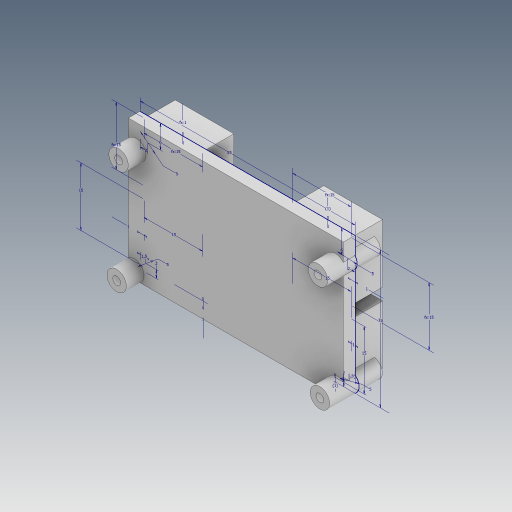
# Autodesk Inventor part: Attacco scheda 2
Saved by Autodesk Inventor 2023.2 (Build 272271000, 271)
## iProperties
Created: 2022-11-27
Part Number: Attacco scheda 2
Material: Generico
Document SubType Name: Modeling
Designer: daler
Density: 1 g/cm^3
Appearance: Default
Author: daler
Autodesk Inventor part; units mm, degrees
ref_plane "YZ Plane" through (0, 0, 0) normal (1, 0, 0) x (0, 1, 0)
ref_plane "XZ Plane" through (0, 0, 0) normal (0, 1, 0) x (-1, 0, 0)
ref_plane "XY Plane" through (0, 0, 0) normal (0, 0, 1) x (1, 0, 0)
sketch "Schizzo1" plane through (0, 0, 0) normal (0, 0, 1) x (1, 0, 0)
  line L0 (-27.5, 17.5) -> (27.5, 17.5)
  line L1 (27.5, 17.5) -> (27.5, -17.5)
  line L2 (27.5, -17.5) -> (-27.5, -17.5)
  line L3 (-27.5, -17.5) -> (-27.5, 17.5)
  line L4 (-27.5, 17.5) -> (27.5, -17.5) construction
  line L5 (27.5, 17.5) -> (-27.5, -17.5) construction
  line L6 (-26.5, 16.5) -> (-11.5, 16.5)
  line L7 (-11.5, 16.5) -> (-11.5, 1.5)
  line L8 (-11.5, 1.5) -> (-26.5, 1.5)
  line L9 (-26.5, 1.5) -> (-26.5, 16.5)
  line L10 (11.5, 16.5) -> (26.5, 16.5)
  line L11 (26.5, 16.5) -> (26.5, 1.5)
  line L12 (26.5, 1.5) -> (11.5, 1.5)
  line L13 (11.5, 1.5) -> (11.5, 16.5)
  line L14 (11.5, -1.5) -> (26.5, -1.5)
  line L15 (26.5, -1.5) -> (26.5, -16.5)
  line L16 (26.5, -16.5) -> (11.5, -16.5)
  line L17 (11.5, -16.5) -> (11.5, -1.5)
  line L18 (-26.5, -1.5) -> (-11.5, -1.5)
  line L19 (-11.5, -1.5) -> (-11.5, -16.5)
  line L20 (-11.5, -16.5) -> (-26.5, -16.5)
  line L21 (-26.5, -16.5) -> (-26.5, -1.5)
  line L22 (-25.5, 17.5) -> (-25.5, 11.5) construction
  line L23 (-25.5, 11.5) -> (-27.5, 11.5) construction
  line L24 (25.5, 17.5) -> (25.5, 11.5) construction
  line L25 (25.5, 11.5) -> (27.5, 11.5) construction
  line L26 (-27.5, -15.5) -> (-26, -15.5) construction
  line L27 (-26, -15.5) -> (-26, -17.5) construction
  line L28 (27.5, -15.5) -> (26, -15.5) construction
  line L29 (26, -15.5) -> (26, -17.5) construction
  circle A0 centre (-25.5, 11.5) radius 2.5
  circle A1 centre (-26, -15.5) radius 2.5
  circle A2 centre (25.5, 11.5) radius 2.5
  circle A3 centre (26, -15.5) radius 2.5
  point P0 (0, 0)
  point P1 (0, 0)
  point P2 (-19, -16.5)
  point P3 (-26.5, -9)
  point P4 (27.5, 13)
  point P5 (-27.5, 13)
  point P6 (-27.5, 10)
  point P7 (-27.5, -13.5)
  point P8 (-24.5, -17.5)
  point P9 (24.5, -17.5)
  point P10 (27.5, -13.5)
  point P11 (27.5, 10)
  dimension "d0" = 55
  dimension "d1" = 35
  dimension "d2" = 15
  dimension "d3" = 15
  dimension "d4" = 1
  dimension "d5" = 1
  dimension "d6" = 15
  dimension "d7" = 15
  dimension "d8" = 1
  dimension "d9" = 15
  dimension "d10" = 15
  dimension "d11" = 1
  dimension "d12" = 1
  dimension "d13" = 15
  dimension "d14" = 1
  dimension "d15" = 15
  dimension "d16" = 1
  dimension "d17" = 6
  dimension "d18" = 2
  dimension "d19" = 6
  dimension "d20" = 2
  dimension "d21" = 1.5
  dimension "d22" = 2
  dimension "d23" = 1.5
  dimension "d24" = 2
  dimension "d25" = 5
  dimension "d26" = 5
  dimension "d27" = 5
  dimension "d28" = 5
  constraints: 60 end point, 12 perpendicular, 11 point on line, 10 parallel, 9 coincident, 6 horizontal, 4 centre point, 3 midpoint
  measures "d0" distance of L0.start L0.end
  measures "d1" distance of L0.end L1.end
  measures "d2" distance of L20.end L18.start
  measures "d3" distance of L18.start L18.end
  measures "d4" distance from line of L2 point (-19, -16.5)
  measures "d5" distance from line of L3 point (-26.5, -9)
  measures "d6" distance of L6.start L6.end
  measures "d7" distance of L8.end L6.start
  measures "d8" distance between parallel lines of L0 L6
  measures "d9" distance of L10.start L10.end
  measures "d10" distance of L10.end L11.end
  measures "d11" distance between parallel lines of L1 L11
  measures "d12" distance between parallel lines of L0 L10
  measures "d13" distance of L14.start L14.end
  measures "d14" distance between parallel lines of L1 L15
  measures "d15" distance of L14.end L15.end
  measures "d16" distance between parallel lines of L2 L16
  measures "d17" distance of L22.start L22.end
  measures "d18" distance of L22.end L23.end
  measures "d19" distance of L24.start L24.end
  measures "d20" distance of L24.end L25.end
  measures "d21" distance of L26.start L26.end
  measures "d22" distance of L26.end L27.end
  measures "d23" distance of L28.start L28.end
  measures "d24" distance of L28.end L29.end
  measures "d25" diameter of A0
  measures "d26" diameter of A1
  measures "d27" diameter of A2
  measures "d28" diameter of A3
extrude "Estrusione1" add sketch "Schizzo1" along normal blind 3
extrude "Estrusione2" add sketch "Schizzo1" against normal blind 8 contours A0 L9 | L9 L6 L7 L8 A0 | A2 L11 L12 L13 L10 | L11 A2 | A1 L20 L21 | L21 L18 L19 L20 A1 | A3 L16 L17 L14 L15 | L15 L16 A3
extrude "Estrusione3" add sketch "Schizzo1" against normal blind 6 contours A0 L9 L3 | L3 A0 | A2 L1 | L1 A2 L11 | A0 L9 | L11 A2 | A1 L21 L20 L2 L3 | L3 A1 | A3 L1 | L1 L2 A3 L16 L15 | L2 A1 | A1 L20 L21 | A3 L2 | L15 L16 A3
hole "Foro1" at (-25.5, 11.5, 0) at (25.5, 11.5, 0) at (-26, -15.5, 0) at (26, -15.5, 0) direction (0, 0, -1) diameter 2 depth 4 tip angle 118 start extended yes
extrude "Estrusione4" add sketch "Schizzo1" along normal blind 7.5 contours A0 L9 L3 | L3 A0 | A2 L1 | L1 A2 L11 | A0 L9 | L11 A2 | A1 L21 L20 L2 L3 | L3 A1 | A3 L1 | L1 L2 A3 L16 L15 | L2 A1 | A1 L20 L21 | A3 L2 | L15 L16 A3
hole "Foro2" at (-25.5, 11.5, 0) at (25.5, 11.5, 0) at (26, -15.5, 0) at (-26, -15.5, 0) direction (0, 0, -1) diameter 2 depth 4 tip angle 118 start extended yes
equation "\"d6\" = d3"
equation "\"d7\" = d2"
equation "\"d8\" = d4"
equation "\"d9\" = d6"
equation "\"d10\" = d9"
